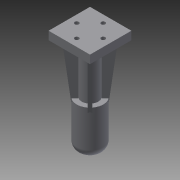
# Autodesk Inventor part: QuadrupedFoot
Saved by Autodesk Inventor 2015 (Build 190159000, 159)
## iProperties
Created: 2015-04-28
Part Number: QuadrupedFoot
Material: ABS Plastic
Document SubType Name: Modeling
Designer: Quinn
Density: 1.06 g/cm^3
Appearance: Smooth - White
Author: Quinn
Autodesk Inventor part; units mm, degrees
ref_plane "YZ Plane" through (0, 0, 0) normal (1, 0, 0) x (0, 1, 0)
ref_plane "XZ Plane" through (0, 0, 0) normal (0, 1, 0) x (-1, 0, 0)
sketch "Sketch2" plane through (0, 0, 0) normal (0, 1, 0) x (-1, 0, 0)
  line L0 (3.940447, 4.971025) -> (-21.059553, 4.971025)
  line L1 (-21.059553, 4.971025) -> (-21.059553, -20.028975)
  line L2 (-21.059553, -20.028975) -> (3.940447, -20.028975)
  line L3 (3.940447, -20.028975) -> (3.940447, 4.971025)
  circle A0 centre (-0.559553, -7.528975) radius 1.25
  circle A1 centre (-16.559553, -7.528975) radius 1.25
  circle A2 centre (-8.559553, 0.471025) radius 1.25
  circle A3 centre (-8.559553, -15.528975) radius 1.25
  point P0 (0, 0)
  dimension "d0" = 25
  dimension "d1" = 25
  dimension "d4" = 2.5
  dimension "d5" = 2.5
  dimension "d8" = 2.5
  dimension "d9" = 2.5
  constraints: 8 end point, 4 centre point, 2 parallel, 1 horizontal, 1 perpendicular
  measures "d0" distance of L2.end L1.end
  measures "d1" distance of L1.end L0.end
  measures "d4" diameter of A0
  measures "d5" diameter of A1
  measures "d8" diameter of A2
  measures "d9" diameter of A3
extrude "Extrusion1" add sketch "Sketch2" along normal blind 7
sketch "Sketch3" plane through (0, 0, 0) normal (0, -1, 0) x (1, 0, 0)
  circle A0 centre (8.559553, -15.528975) radius 1.25
  circle A1 centre (8.559553, 0.471025) radius 1.25
  circle A2 centre (16.559553, -7.528975) radius 1.25
  circle A3 centre (0.559553, -7.528975) radius 1.25
  line L0 (-3.940447, 4.971025) -> (21.059553, 4.971025)
  line L1 (-3.940447, -20.028975) -> (-3.940447, 4.971025)
  line L2 (21.059553, -20.028975) -> (-3.940447, -20.028975)
  line L3 (21.059553, 4.971025) -> (21.059553, -20.028975)
  circle A4 centre (8.559553, -7.528975) radius 5
  point P0 (0, 0)
  dimension "d12" = 10
  constraints: 1 centre point
  measures "d12" diameter of A4
extrude "Extrusion2" add sketch "Sketch3" along normal blind 55 contours A4
sketch "Sketch4" plane through (0, 0, 0) normal (0, -1, 0) x (1, 0, 0)
  circle A0 centre (8.559553, -7.528975) radius 5
  circle A1 centre (8.559553, -15.528975) radius 1.25
  circle A2 centre (8.559553, 0.471025) radius 1.25
  circle A3 centre (16.559553, -7.528975) radius 1.25
  circle A4 centre (0.559553, -7.528975) radius 1.25
  line L0 (-3.940447, 4.971025) -> (21.059553, 4.971025)
  line L1 (-3.940447, -20.028975) -> (-3.940447, 4.971025)
  line L2 (21.059553, -20.028975) -> (-3.940447, -20.028975)
  line L3 (21.059553, 4.971025) -> (21.059553, -20.028975)
  circle A5 centre (8.559553, -15.528975) radius 2.25
  circle A6 centre (16.559553, -7.528975) radius 2.25
  circle A7 centre (8.559553, 0.471025) radius 2.25
  circle A8 centre (0.559553, -7.528975) radius 2.25
  point P0 (0, 0)
  dimension "d15" = 1
  dimension "d16" = 1
  dimension "d17" = 1
  dimension "d18" = 1
  constraints: 4 centre point
  measures "d15" radial gap between concentric circles of A1 A5
  measures "d16" radial gap between concentric circles of A3 A6
  measures "d17" radial gap between concentric circles of A2 A7
  measures "d18" radial gap between concentric circles of A4 A8
extrude "Extrusion3" cut sketch "Sketch4" against normal blind 2 contours A5 | A6 | A7 | A8
ref_plane "Work Plane1" through (-3.940447, 0, -20.028975) normal (-0.7071068, 0, 0.7071068) x (0, 1, 0)
sketch "Sketch6" plane through (-3.940447, 0, -20.028975) normal (-0.7071068, 0, 0.7071068) x (0, 1, 0)
  line L0 (-55, -12.67767) -> (-55, -22.67767)
  line L1 (0, -22.67767) -> (0, -12.67767)
  line L2 (0, -12.67767) -> (-55, -12.67767)
  line L3 (0, -25.584524) -> (0, -21.084524)
  line L4 (0, -14.270815) -> (0, -9.770815)
  line L5 (0, -25.584524) -> (0, -21.084524)
  line L6 (0, -14.270815) -> (0, -9.770815)
  line L7 (0, -22.67767) -> (0, -12.67767)
  line L8 (0, -17.67767) -> (0, -35.355339)
  line L9 (0, 0) -> (0, -17.67767)
  line L10 (0, -17.67767) -> (0, 0)
  line L11 (0, -35.355339) -> (0, -17.67767)
  line L12 (-55, -12.67767) -> (0, -6.083473)
  line L13 (0, -6.083473) -> (0, -12.67767)
  line L14 (-55, -12.67767) -> (0, -12.67767)
  point P0 (0, -16.948941)
  constraints: 6 end point, 2 collinear, 1 point on line
extrude "Extrusion4" add sketch "Sketch6" along normal mid plane 2
pattern_circular "Circular Pattern1" count 4 over 360 about axis through (8.559553, 0, -7.528975) along (0, -1, 0) of "Extrusion4"
sketch "Sketch7" plane through (0, -55, 0) normal (0, -1, 0) x (1, 0, 0)
  arc A0 (5.024019, -11.064509) -> (12.095087, -11.064509) centre (8.559553, -7.528975) ccw
  arc A1 (12.095087, -11.064509) -> (12.095087, -3.993441) centre (8.559553, -7.528975) ccw
  arc A2 (12.095087, -3.993441) -> (5.024019, -3.993441) centre (8.559553, -7.528975) ccw
  arc A3 (5.024019, -3.993441) -> (5.024019, -11.064509) centre (8.559553, -7.528975) ccw
  arc A4 (14.216407, -13.185829) -> (14.216407, -1.87212) centre (8.559553, -7.528975) ccw
  arc A5 (2.902699, -13.185829) -> (14.216407, -13.185829) centre (8.559553, -7.528975) ccw
  arc A6 (2.902699, -1.87212) -> (2.902699, -13.185829) centre (8.559553, -7.528975) ccw
  arc A7 (14.216407, -1.87212) -> (2.902699, -1.87212) centre (8.559553, -7.528975) ccw
  point P0 (0, 0)
  dimension "d26" = 3
  constraints: 8 point on circle, 4 centre point, 3 other
  measures "d26" radial gap between concentric circles of A1 A4
extrude "Extrusion5" add sketch "Sketch7" against normal blind 27.4
fillet "Fillet1" radius 5.175 1 edges at (14.2164, -55, -1.8721)
chamfer "Chamfer1" distance 2 angle 45 4 edges at (21.0596, 0, -7.529) (8.5596, 0, -20.029) (-3.9404, 0, -7.529) (8.5596, 0, 4.971)
body "Solid1"
